Autodesk Fusion 360 part; units mm, degrees
note: some values were not read from the file. Set by a fixed rule: which face or edge a step refers to.
(part 2 of 2)
sketch "Sketch35" plane through (0, 0, 28.5) normal (0, 0, -1) x (1, 0, 0)
  line L0 (-117.5, -71.5) -> (117.5, -71.5)
  line L1 (117.5, -71.5) -> (117.5, -22.5)
  line L2 (117.5, -22.5) -> (117.5, 22.5)
  line L3 (117.5, 22.5) -> (117.5, 74)
  line L4 (117.5, 74) -> (-117.5, 74)
  line L5 (-117.5, 74) -> (-117.5, 22.5)
  line L6 (-117.5, 22.5) -> (-117.5, -22.5)
  line L7 (-117.5, -22.5) -> (-117.5, -71.5)
  line L8 (122.5, -76.5) -> (122.5, 79)
  circle A0 centre (29.5, 1.25) radius 4
  line L9 (0, 94.55) -> (0, -92.05)
  circle A1 centre (-29.5, 1.25) radius 4
  line L10 (117.5, -71.5) -> (-117.5, -71.5)
  line L11 (117.5, -71.5) -> (117.5, -22.5)
  line L12 (77.3093, -22.5) -> (77.3093, -71.5)
  line L13 (77.3093, -71.5) -> (117.5, -71.5)
  line L14 (117.5, -71.5) -> (117.5, -22.5)
  line L15 (77.3093, -71.5) -> (69.4734, -65.0728)
  line L16 (-105, 30) -> (-100, 30)
  line L17 (-100, 30) -> (-100, -45)
  line L18 (-100, -45) -> (-105, -45)
  line L19 (-105, -45) -> (-105, 30)
  line L20 (-95, 30) -> (-90, 30)
  line L21 (-90, 30) -> (-90, -45)
  line L22 (-90, -45) -> (-95, -45)
  line L23 (-95, -45) -> (-95, 30)
  line L24 (-85, 30) -> (-80, 30)
  line L25 (-80, 30) -> (-80, -45)
  line L26 (-80, -45) -> (-85, -45)
  line L27 (-85, -45) -> (-85, 30)
  line L28 (-75, 30) -> (-70, 30)
  line L29 (-70, 30) -> (-70, -45)
  line L30 (-70, -45) -> (-75, -45)
  line L31 (-75, -45) -> (-75, 30)
  line L32 (-65, 30) -> (-60, 30)
  line L33 (-60, 30) -> (-60, -45)
  line L34 (-60, -45) -> (-65, -45)
  line L35 (-65, -45) -> (-65, 30)
  line L36 (75, -45) -> (75, 30)
  line L37 (70, 30) -> (70, -45)
  line L38 (100, -45) -> (105, -45)
  line L39 (90, -45) -> (95, -45)
  line L40 (65, -45) -> (65, 30)
  line L41 (85, -45) -> (85, 30)
  line L42 (70, -45) -> (75, -45)
  line L43 (105, -45) -> (105, 30)
  line L44 (95, 30) -> (90, 30)
  line L45 (80, 30) -> (80, -45)
  line L46 (60, 30) -> (60, -45)
  line L47 (90, 30) -> (90, -45)
  line L48 (85, 30) -> (80, 30)
  line L49 (100, 30) -> (100, -45)
  line L50 (75, 30) -> (70, 30)
  line L51 (65, 30) -> (60, 30)
  line L52 (95, -45) -> (95, 30)
  line L53 (60, -45) -> (65, -45)
  line L54 (80, -45) -> (85, -45)
  line L55 (105, 30) -> (100, 30)
  dimension "d201" = 8
  constraint symmetric A0 L9 A1
  constraint coincident L10 L12.end
  constraint coincident L1.end L2.start
  constraint vertical L12
  constraint horizontal L13
  constraint vertical L14
  constraint horizontal L16
  constraint vertical L17
  constraint horizontal L18
  constraint vertical L19
  constraint horizontal L20
  constraint vertical L21
  constraint horizontal L22
  constraint vertical L23
  constraint horizontal L24
  constraint vertical L25
  constraint horizontal L26
  constraint vertical L27
  constraint horizontal L28
  constraint vertical L29
  constraint horizontal L30
  constraint vertical L31
  constraint horizontal L32
  constraint vertical L33
  constraint horizontal L34
  constraint vertical L35
  constraint symmetric L9 L16.start L43.end
  constraint symmetric L9 L16.end L49.start
  constraint symmetric L9 L17.end L38.start
  constraint symmetric L9 L18.end L38.end
  constraint symmetric L9 L20.start L44.start
  constraint symmetric L9 L20.end L44.end
  constraint symmetric L9 L21.end L39.start
  constraint symmetric L9 L22.end L39.end
  constraint symmetric L9 L24.start L41.end
  constraint symmetric L9 L24.end L45.start
  constraint symmetric L9 L25.end L45.end
  constraint symmetric L9 L26.end L41.start
  constraint symmetric L9 L28.start L36.end
  constraint symmetric L9 L28.end L37.start
  constraint symmetric L9 L29.end L37.end
  constraint symmetric L9 L30.end L36.start
  constraint symmetric L9 L32.start L40.end
  constraint symmetric L9 L32.end L46.start
  constraint symmetric L9 L33.end L46.end
  constraint symmetric L9 L34.end L40.start
  measures "d201" diameter of A0
extrude "Extrude59" cut sketch "Sketch35" against normal blind 50 contours A0 | A1 | L16 L17 L18 L19 | L20 L21 L22 L23 | L24 L25 L26 L27 | L28 L29 L30 L31 | L32 L33 L34 L35 | L36 L37 L42 L50 | L38 L43 L49 L55 | L39 L44 L47 L52 | L40 L46 L51 L53 | L41 L45 L48 L54 bodies 4
sketch "Sketch36" plane through (0, 0, 28.5) normal (0, 0, -1) x (1, 0, 0)
  line L0 (-80, 30) -> (-80, -45)
  line L1 (-80, -45) -> (-85, -45)
  line L2 (-85, -45) -> (-85, 30)
  line L3 (-85, 30) -> (-80, 30)
  circle A0 centre (29.5, 1.25) radius 4
  line L4 (70, -45) -> (70, 30)
  line L5 (70, 30) -> (75, 30)
  line L6 (75, 30) -> (75, -45)
  line L7 (75, -45) -> (70, -45)
  line L8 (85, 30) -> (85, -45)
  line L9 (85, -45) -> (80, -45)
  line L10 (80, -45) -> (80, 30)
  line L11 (80, 30) -> (85, 30)
  circle A1 centre (-29.5, 1.25) radius 4
  line L12 (-90, 30) -> (-90, -45)
  line L13 (-90, -45) -> (-95, -45)
  line L14 (-95, -45) -> (-95, 30)
  line L15 (-95, 30) -> (-90, 30)
  line L16 (-70, 30) -> (-70, -45)
  line L17 (-70, -45) -> (-75, -45)
  line L18 (-75, -45) -> (-75, 30)
  line L19 (-75, 30) -> (-70, 30)
  line L20 (100, -45) -> (100, 30)
  line L21 (100, 30) -> (105, 30)
  line L22 (105, 30) -> (105, -45)
  line L23 (105, -45) -> (100, -45)
  line L24 (65, 30) -> (65, -45)
  line L25 (65, -45) -> (60, -45)
  line L26 (60, -45) -> (60, 30)
  line L27 (60, 30) -> (65, 30)
  line L28 (90, 30) -> (95, 30)
  line L29 (95, 30) -> (95, -45)
  line L30 (95, -45) -> (90, -45)
  line L31 (90, -45) -> (90, 30)
  line L32 (-60, 30) -> (-60, -45)
  line L33 (-60, -45) -> (-65, -45)
  line L34 (-65, -45) -> (-65, 30)
  line L35 (-65, 30) -> (-60, 30)
  line L36 (-100, 30) -> (-100, -45)
  line L37 (-100, -45) -> (-105, -45)
  line L38 (-105, -45) -> (-105, 30)
  line L39 (-105, 30) -> (-100, 30)
  line L40 (-117.5, -71.5) -> (117.5, -71.5)
  line L41 (117.5, -71.5) -> (117.5, -22.5)
  line L42 (117.5, -22.5) -> (117.5, 22.5)
  line L43 (117.5, 22.5) -> (117.5, 74)
  line L44 (117.5, 74) -> (-117.5, 74)
  line L45 (-117.5, 74) -> (-117.5, 22.5)
  line L46 (-117.5, 22.5) -> (-117.5, -22.5)
  line L47 (-117.5, -22.5) -> (-117.5, -71.5)
  circle A2 centre (29.5, 1.25) radius 4
  circle A3 centre (-29.5, 1.25) radius 4
  circle A4 centre (-29.5, 1.25) radius 4.5
  circle A5 centre (29.5, 1.25) radius 4.5
  dimension "d204" = 9
  dimension "d205" = 9
  constraint concentric A3 A4
  constraint concentric A2 A5
  measures "d204" diameter of A4
  measures "d205" diameter of A5
extrude "Extrude60" cut sketch "Sketch36" against normal blind 45 contours A0 A2 | A4 bodies 4
extrude "Extrude61" cut 1 faces at (122.5, -27.1667, 39.3333) along direction (-1, 0, 0) blind 2.5 on bodies 4 bodies 4
extrude "Extrude62" cut 1 faces at (-122.5, 24.6667, 39.3333) along direction (1, 0, 0) blind 2.5 on bodies 4 bodies 4
split "Split8" by plane through (0, -1.25, 18.25) normal (1, 0, 0) bodies 4 makes body 6 at (60, -62.6667, 45)
sketch "Sketch37" plane through (0, 0, 0) normal (1, 0, 0) x (0, 1, 0)
  line L0 (-74, 36.5) -> (-74, 28.5)
  line L1 (-74, 28.5) -> (71.5, 28.5)
  line L2 (71.5, 28.5) -> (71.5, 36.5)
  line L3 (71.5, 36.5) -> (76.5, 36.5)
  line L4 (76.5, 36.5) -> (76.5, 45)
  line L5 (76.5, 45) -> (-79, 45)
  line L6 (-79, 45) -> (-79, 36.5)
  line L7 (-79, 36.5) -> (-74, 36.5)
  line L8 (0, 45) -> (0, 28.5)
  line L9 (30, 31.75) -> (-30, 31.75)
  line L10 (-30, 31.75) -> (-30, 41.75)
  line L11 (-30, 41.75) -> (30, 41.75)
  line L12 (30, 41.75) -> (30, 31.75)
  line L13 (30, 31.75) -> (-30, 41.75) construction
  line L14 (-30, 31.75) -> (30, 41.75) construction
  point P0 (0, 36.75)
  dimension "d212" = 60
  dimension "d213" = 10
  constraint coincident L5 L8.start
  constraint coincident L1 L8.end
  constraint perpendicular L1 L8
  constraint horizontal L9
  constraint perpendicular L9 L10
  constraint parallel L9 L11
  constraint parallel L10 L12
  constraint coincident L13 P0
  constraint coincident L14 P0
  constraint midpoint L8 P0
  measures "d212" distance of L10.end L11.end
  measures "d213" distance of L9.end L10.end
extrude "Extrude63" add sketch "Sketch37" along normal blind 20 draft -45 contours L8 L9 L10 L11 | L8 L9 L11 L12 bodies 4
sketch "Sketch38" plane through (0, 0, 0) normal (-1, 0, 0) x (0, -1, 0)
  line L0 (74, 28.5) -> (74, 36.5)
  line L1 (74, 36.5) -> (79, 36.5)
  line L2 (79, 36.5) -> (79, 45)
  line L3 (79, 45) -> (-76.5, 45)
  line L4 (-76.5, 45) -> (-76.5, 36.5)
  line L5 (-76.5, 36.5) -> (-71.5, 36.5)
  line L6 (-71.5, 36.5) -> (-71.5, 28.5)
  line L7 (-71.5, 28.5) -> (74, 28.5)
  line L8 (30, 31.75) -> (30, 41.75)
  line L9 (-30, 31.75) -> (30, 31.75)
  line L10 (30, 41.75) -> (-30, 41.75)
  line L11 (-30, 41.75) -> (-30, 31.75)
extrude "Extrude64" cut sketch "Sketch38" against normal blind 10 draft -45 contours L8 L9 L10 L11 bodies 6
sketch "Sketch39" plane through (0, 0, 45) normal (0, 0, 1) x (-1, 0, 0)
  line L0 (0, 79) -> (0, -76.5)
  line L1 (0, -76.5) -> (120, -76.5)
  line L2 (120, -76.5) -> (120, 79)
  line L3 (120, 79) -> (0, 79)
  circle A0 centre (29.5, 1.25) radius 4.5
  line L4 (80, -45) -> (80, 30)
  line L5 (80, 30) -> (85, 30)
  line L6 (85, 30) -> (85, -45)
  line L7 (85, -45) -> (80, -45)
  line L8 (90, -45) -> (90, 30)
  line L9 (90, 30) -> (95, 30)
  line L10 (95, 30) -> (95, -45)
  line L11 (95, -45) -> (90, -45)
  line L12 (70, -45) -> (70, 30)
  line L13 (70, 30) -> (75, 30)
  line L14 (75, 30) -> (75, -45)
  line L15 (75, -45) -> (70, -45)
  line L16 (60, -45) -> (60, 30)
  line L17 (60, 30) -> (65, 30)
  line L18 (65, 30) -> (65, -45)
  line L19 (65, -45) -> (60, -45)
  line L20 (100, -45) -> (100, 30)
  line L21 (100, 30) -> (105, 30)
  line L22 (105, 30) -> (105, -45)
  line L23 (105, -45) -> (100, -45)
sketch "Sketch40" plane through (0, 0, 45) normal (0, 0, 1) x (-1, 0, 0)
  line L0 (0, 79) -> (0, -76.5)
  line L1 (0, -76.5) -> (120, -76.5)
  line L2 (120, -76.5) -> (120, 79)
  line L3 (120, 79) -> (0, 79)
  circle A0 centre (29.5, 1.25) radius 4.5
  line L4 (80, -45) -> (80, 30)
  line L5 (80, 30) -> (85, 30)
  line L6 (85, 30) -> (85, -45)
  line L7 (85, -45) -> (80, -45)
  line L8 (90, -45) -> (90, 30)
  line L9 (90, 30) -> (95, 30)
  line L10 (95, 30) -> (95, -45)
  line L11 (95, -45) -> (90, -45)
  line L12 (70, -45) -> (70, 30)
  line L13 (70, 30) -> (75, 30)
  line L14 (75, 30) -> (75, -45)
  line L15 (75, -45) -> (70, -45)
  line L16 (60, -45) -> (60, 30)
  line L17 (60, 30) -> (65, 30)
  line L18 (65, 30) -> (65, -45)
  line L19 (65, -45) -> (60, -45)
  line L20 (100, -45) -> (100, 30)
  line L21 (100, 30) -> (105, 30)
  line L22 (105, 30) -> (105, -45)
  line L23 (105, -45) -> (100, -45)
  line L24 (30, -50) -> (35, -50)
  line L25 (35, -50) -> (35, -63)
  line L26 (35, -63) -> (30, -63)
  line L27 (30, -63) -> (30, -50)
  line L28 (0, 0) -> (20, 0)
  line L29 (30, 63) -> (30, 50)
  line L30 (35, 63) -> (30, 63)
  line L31 (30, 50) -> (35, 50)
  line L32 (35, 50) -> (35, 63)
  dimension "d218" = 5
  dimension "d219" = 13
  constraint horizontal L24
  constraint vertical L25
  constraint horizontal L26
  constraint vertical L27
  constraint coincident L28.start origin
  constraint perpendicular L0 L28
  constraint symmetric L24.start L28 L29.end
  constraint symmetric L24.end L28 L31.end
  constraint symmetric L25.end L28 L30.start
  constraint symmetric L26.end L28 L29.start
  measures "d218" distance of L24.start L24.end
  measures "d219" distance of L24.start L26.end
extrude "Extrude65" cut sketch "Sketch40" against normal blind 20 contours L24 L25 L26 L27 bodies 4
mirror "Mirror11" about plane through (0, 0, 0) normal (0, 1, 0) of "Extrude65"
sketch "Sketch41" plane through (0, 0, 45) normal (0, 0, 1) x (-1, 0, 0)
  line L0 (0, -76.5) -> (0, 79)
  line L1 (0, 79) -> (-120, 79)
  line L2 (-120, 79) -> (-120, -76.5)
  line L3 (-120, -76.5) -> (0, -76.5)
  line L4 (-95, 30) -> (-90, 30)
  line L5 (-90, 30) -> (-90, -45)
  line L6 (-90, -45) -> (-95, -45)
  line L7 (-95, -45) -> (-95, 30)
  line L8 (-65, -45) -> (-65, 30)
  line L9 (-65, 30) -> (-60, 30)
  line L10 (-60, 30) -> (-60, -45)
  line L11 (-60, -45) -> (-65, -45)
  line L12 (-100, 30) -> (-100, -45)
  line L13 (-100, -45) -> (-105, -45)
  line L14 (-105, -45) -> (-105, 30)
  line L15 (-105, 30) -> (-100, 30)
  line L16 (-85, -45) -> (-85, 30)
  line L17 (-85, 30) -> (-80, 30)
  line L18 (-80, 30) -> (-80, -45)
  line L19 (-80, -45) -> (-85, -45)
  line L20 (-70, 30) -> (-70, -45)
  line L21 (-70, -45) -> (-75, -45)
  line L22 (-75, -45) -> (-75, 30)
  line L23 (-75, 30) -> (-70, 30)
  circle A0 centre (-29.5, 1.25) radius 4
  line L24 (30, -50) -> (35, -50)
  line L25 (35, -63) -> (30, -63)
  line L26 (0, 79) -> (0, 50)
  line L27 (-30, -50) -> (-35, -50)
  line L28 (-35, -63) -> (-30, -63)
  line L29 (-35, -50) -> (-30, -50)
  line L30 (-30, -50) -> (-30, -63)
  line L31 (-30, -63) -> (-35, -63)
  line L32 (-35, -63) -> (-35, -50)
  constraint coincident L0.end L1.start
  constraint coincident L0 L26.end
  constraint symmetric L24.start L26 L27.start
  constraint symmetric L24.end L26 L27.end
  constraint symmetric L25.start L26 L28.start
  constraint symmetric L25.end L26 L28.end
  constraint horizontal L29
  constraint vertical L30
  constraint horizontal L31
  constraint vertical L32
extrude "Extrude66" cut sketch "Sketch41" against normal blind 25 contours L27 L28 L29 L30 L31 L32 bodies 6
mirror "Mirror12" about plane through (0, 0, 0) normal (0, 1, 0) of "Extrude66"
sketch "Sketch42" plane through (0, 0, 28.5) normal (0, 0, -1) x (1, 0, 0)
  line L0 (30, 50) -> (30, 63)
  line L1 (30, 63) -> (35, 63)
  line L2 (35, 63) -> (35, 50)
  line L3 (35, 50) -> (30, 50)
  line L4 (30, -63) -> (30, -50)
  line L5 (30, -50) -> (35, -50)
  line L6 (35, -50) -> (35, -63)
  line L7 (35, -63) -> (30, -63)
  line L8 (0, 74) -> (0, -71.5)
  line L9 (0, -71.5) -> (117.5, -71.5)
  line L10 (117.5, -71.5) -> (117.5, -22.5)
  line L11 (117.5, -22.5) -> (117.5, 22.5)
  line L12 (117.5, 22.5) -> (117.5, 74)
  line L13 (117.5, 74) -> (0, 74)
  circle A0 centre (29.5, 1.25) radius 4
  line L14 (70, -45) -> (70, 30)
  line L15 (70, 30) -> (75, 30)
  line L16 (75, 30) -> (75, -45)
  line L17 (75, -45) -> (70, -45)
  line L18 (85, 30) -> (85, -45)
  line L19 (85, -45) -> (80, -45)
  line L20 (80, -45) -> (80, 30)
  line L21 (80, 30) -> (85, 30)
  line L22 (100, -45) -> (100, 30)
  line L23 (100, 30) -> (105, 30)
  line L24 (105, 30) -> (105, -45)
  line L25 (105, -45) -> (100, -45)
  line L26 (65, 30) -> (65, -45)
  line L27 (65, -45) -> (60, -45)
  line L28 (60, -45) -> (60, 30)
  line L29 (60, 30) -> (65, 30)
  line L30 (90, 30) -> (95, 30)
  line L31 (95, 30) -> (95, -45)
  line L32 (95, -45) -> (90, -45)
  line L33 (90, -45) -> (90, 30)
  line L34 (110, -64) -> (110, -22.5)
  line L35 (110, -22.5) -> (110, 22.5)
  line L36 (110, 22.5) -> (110, 66.5)
  line L37 (110, 66.5) -> (7.5, 66.5)
  line L38 (7.5, -64) -> (110, -64)
  line L39 (7.5, 66.5) -> (0, 66.5)
  line L40 (7.5, -64) -> (0, -64)
  dimension "d228" = -7.5
  constraint coincident L8 L39.end
  constraint perpendicular L8 L39
  constraint coincident L8 L40.end
  constraint perpendicular L8 L40
extrude "Extrude67" cut sketch "Sketch42" against normal up to surface (8 mm away) contours L8 L34 L35 L36 L37 L38 L39 L40 bodies 4 6
sketch "Sketch43" plane through (0, 0, 28.5) normal (0, 0, -1) x (1, 0, 0)
  line L0 (-35, 50) -> (-35, 63)
  line L1 (-35, 63) -> (-30, 63)
  line L2 (-30, 63) -> (-30, 50)
  line L3 (-30, 50) -> (-35, 50)
  line L4 (-35, -63) -> (-35, -50)
  line L5 (-35, -50) -> (-30, -50)
  line L6 (-30, -50) -> (-30, -63)
  line L7 (-30, -63) -> (-35, -63)
  line L8 (0, -71.5) -> (0, 74)
  line L9 (0, 74) -> (-117.5, 74)
  line L10 (-117.5, 74) -> (-117.5, 22.5)
  line L11 (-117.5, 22.5) -> (-117.5, -22.5)
  line L12 (-117.5, -22.5) -> (-117.5, -71.5)
  line L13 (-117.5, -71.5) -> (0, -71.5)
  line L14 (-100, 30) -> (-100, -45)
  line L15 (-100, -45) -> (-105, -45)
  line L16 (-105, -45) -> (-105, 30)
  line L17 (-105, 30) -> (-100, 30)
  line L18 (-60, 30) -> (-60, -45)
  line L19 (-60, -45) -> (-65, -45)
  line L20 (-65, -45) -> (-65, 30)
  line L21 (-65, 30) -> (-60, 30)
  line L22 (-70, 30) -> (-70, -45)
  line L23 (-70, -45) -> (-75, -45)
  line L24 (-75, -45) -> (-75, 30)
  line L25 (-75, 30) -> (-70, 30)
  line L26 (-90, 30) -> (-90, -45)
  line L27 (-90, -45) -> (-95, -45)
  line L28 (-95, -45) -> (-95, 30)
  line L29 (-95, 30) -> (-90, 30)
  line L30 (-80, 30) -> (-80, -45)
  line L31 (-80, -45) -> (-85, -45)
  line L32 (-85, -45) -> (-85, 30)
  line L33 (-85, 30) -> (-80, 30)
  circle A0 centre (-29.5, 1.25) radius 4.5
  line L34 (0, 66.5) -> (110, 66.5)
  line L35 (110, 66.5) -> (110, -64)
  line L36 (110, -64) -> (0, -64)
  line L37 (0, -64) -> (0, -71.5)
  line L38 (0, -71.5) -> (117.5, -71.5)
  line L39 (117.5, -71.5) -> (117.5, -22.5)
  line L40 (117.5, -22.5) -> (117.5, 22.5)
  line L41 (117.5, 22.5) -> (117.5, 74)
  line L42 (117.5, 74) -> (0, 74)
  line L43 (0, 74) -> (0, 66.5)
  line L44 (0, 66.5) -> (-110, 66.5)
  line L45 (-110, 66.5) -> (-110, -64)
  line L46 (-110, -64) -> (0, -64)
  constraint symmetric L8 L34.start L43.end
  constraint symmetric L8 L34.end L44.end
  constraint symmetric L8 L35.end L45.end
  constraint symmetric L8 L36.end L37.start
extrude "Extrude68" cut sketch "Sketch43" against normal up to surface (8 mm away) contours L8 L44 L45 L46 bodies 4
sketch "Sketch44" plane through (0, 0, 0) normal (1, 0, 0) x (0, 1, 0)
  line L0 (64, 36.5) -> (64, 28.5)
  line L1 (64, 28.5) -> (71.5, 28.5)
  line L2 (71.5, 28.5) -> (71.5, 36.5)
  line L3 (71.5, 36.5) -> (76.5, 36.5)
  line L4 (76.5, 36.5) -> (76.5, 45)
  line L5 (76.5, 45) -> (-79, 45)
  line L6 (-79, 45) -> (-79, 36.5)
  line L7 (-79, 36.5) -> (-74, 36.5)
  line L8 (-74, 36.5) -> (-74, 28.5)
  line L9 (-74, 28.5) -> (-66.5, 28.5)
  line L10 (-66.5, 28.5) -> (-66.5, 36.5)
  line L11 (-66.5, 36.5) -> (-30, 36.5)
  line L12 (-30, 36.5) -> (-30, 41.75)
  line L13 (-30, 41.75) -> (30, 41.75)
  line L14 (30, 41.75) -> (30, 36.5)
  line L15 (30, 36.5) -> (64, 36.5)
  line L16 (-30, 41.75) -> (30, 41.75)
  line L17 (30, 41.75) -> (30, 36.5)
  line L18 (30, 36.5) -> (-30, 36.5)
  line L19 (-30, 36.5) -> (-30, 41.75)
  point P0 (-30, 41.75)
  constraint horizontal L16
  constraint vertical L17
  constraint horizontal L18
  constraint vertical L19
  constraint coincident L14.end L15.start
  constraint coincident P0 L12.end
extrude "Extrude69" cut sketch "Sketch44" along normal blind 24 bodies 4
sketch "Sketch45" plane through (0, 0, 0) normal (1, 0, 0) x (0, 1, 0)
  line L0 (64, 36.5) -> (64, 28.5)
  line L1 (64, 28.5) -> (71.5, 28.5)
  line L2 (71.5, 28.5) -> (71.5, 36.5)
  line L3 (71.5, 36.5) -> (76.5, 36.5)
  line L4 (76.5, 36.5) -> (76.5, 45)
  line L5 (76.5, 45) -> (-79, 45)
  line L6 (-79, 45) -> (-79, 36.5)
  line L7 (-79, 36.5) -> (-74, 36.5)
  line L8 (-74, 36.5) -> (-74, 28.5)
  line L9 (-74, 28.5) -> (-66.5, 28.5)
  line L10 (-66.5, 28.5) -> (-66.5, 36.5)
  line L11 (-66.5, 36.5) -> (64, 36.5)
  line L12 (25, 38.25) -> (-25, 38.25)
  line L13 (-25, 38.25) -> (-25, 43.25)
  line L14 (-25, 43.25) -> (25, 43.25)
  line L15 (25, 43.25) -> (25, 38.25)
  line L16 (25, 38.25) -> (-25, 43.25) construction
  line L17 (-25, 38.25) -> (25, 43.25) construction
  point P0 (0, 40.75)
  dimension "d235" = 8.5
  dimension "d236" = 50
  dimension "d237" = 5
  dimension "d238" = 4.25
  constraint horizontal L12
  constraint perpendicular L12 L13
  constraint parallel L12 L14
  constraint parallel L13 L15
  constraint coincident L16 P0
  constraint coincident L17 P0
  measures "d235" distance of L5.end L6.end
  measures "d236" distance of L13.end L14.end
  measures "d237" distance of L12.end L13.end
  measures "d238" vertical distance of L6.end P0
extrude "Extrude70" add sketch "Sketch45" along normal blind 45 draft -45 contours L12 L13 L14 L15 bodies 4
sketch "Sketch46" plane through (0, 0, 0) normal (-1, 0, 0) x (0, -1, 0)
  line L0 (66.5, 36.5) -> (66.5, 28.5)
  line L1 (66.5, 28.5) -> (74, 28.5)
  line L2 (74, 28.5) -> (74, 36.5)
  line L3 (74, 36.5) -> (79, 36.5)
  line L4 (79, 36.5) -> (79, 45)
  line L5 (79, 45) -> (-76.5, 45)
  line L6 (-76.5, 45) -> (-76.5, 36.5)
  line L7 (-76.5, 36.5) -> (-71.5, 36.5)
  line L8 (-71.5, 36.5) -> (-71.5, 28.5)
  line L9 (-71.5, 28.5) -> (-64, 28.5)
  line L10 (-64, 28.5) -> (-64, 36.5)
  line L11 (-64, 36.5) -> (-30, 36.5)
  line L12 (-30, 36.5) -> (-30, 41.75)
  line L13 (-30, 41.75) -> (30, 41.75)
  line L14 (30, 41.75) -> (30, 36.5)
  line L15 (30, 36.5) -> (66.5, 36.5)
  line L16 (-30, 41.75) -> (30, 41.75)
  line L17 (30, 41.75) -> (30, 36.5)
  line L18 (30, 36.5) -> (-30, 36.5)
  line L19 (-30, 36.5) -> (-30, 41.75)
  constraint horizontal L16
  constraint vertical L17
  constraint horizontal L18
  constraint vertical L19
  constraint coincident L14.end L15.start
  constraint coincident L12.end L13.start
extrude "Extrude71" add sketch "Sketch46" against normal blind 10 contours L12 L13 L14 L16 L17 L18 L19 bodies 6
sketch "Sketch47" plane through (0, 0, 0) normal (-1, 0, 0) x (0, -1, 0)
  line L0 (66.5, 36.5) -> (66.5, 28.5)
  line L1 (66.5, 28.5) -> (74, 28.5)
  line L2 (74, 28.5) -> (74, 36.5)
  line L3 (74, 36.5) -> (79, 36.5)
  line L4 (79, 36.5) -> (79, 45)
  line L5 (79, 45) -> (-76.5, 45)
  line L6 (-76.5, 45) -> (-76.5, 36.5)
  line L7 (-76.5, 36.5) -> (-71.5, 36.5)
  line L8 (-71.5, 36.5) -> (-71.5, 28.5)
  line L9 (-71.5, 28.5) -> (-64, 28.5)
  line L10 (-64, 28.5) -> (-64, 36.5)
  line L11 (-64, 36.5) -> (66.5, 36.5)
  line L12 (25, 43.25) -> (-25, 43.25)
  line L13 (-25, 38.25) -> (25, 38.25)
  line L14 (-25, 43.25) -> (25, 43.25)
  line L15 (25, 43.25) -> (25, 38.25)
  line L16 (25, 38.25) -> (-25, 38.25)
  line L17 (-25, 38.25) -> (-25, 43.25)
  constraint horizontal L14
  constraint vertical L15
  constraint horizontal L16
  constraint vertical L17
  constraint coincident L13.end L15.end
  constraint coincident L12.end L14.start
extrude "Extrude72" cut sketch "Sketch47" against normal blind 25 draft -45 contours L12 L13 L14 L15 L16 L17 bodies 6
equation "d238 = ( 8.50 / 2 ) * 1 mm"
named bodies: "Half2", "Half1", "backplate", "backplate (1)"
